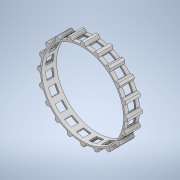
# Autodesk Inventor part: tracks_v1
Saved by Autodesk Inventor 2020 (Build 240168000, 168)
## iProperties
Created: 2020-04-20
Part Number: tracks_v1
Material: Ogólny
Document SubType Name: Modeling
Designer: blep
Density: 1 g/cm^3
Appearance: Domyślna
Author: blep
Autodesk Inventor part; units mm, degrees
ref_plane "XZ Plane" through (0, 0, 0) normal (0, 1, 0) x (-1, 0, 0)
ref_plane "XY Plane" through (0, 0, 0) normal (0, 0, 1) x (1, 0, 0)
sketch "Szkic1" plane through (0, 0, 0) normal (0, 0, 1) x (1, 0, 0)
  circle A0 centre (0, 0) radius 55.5545
  circle A1 centre (0, 0) radius 57.5545
  dimension "d0" = 111.109
  dimension "d1" = 2
  constraints: 2 centre point, 1 coincident
  measures "d0" diameter of A0
  measures "d1" radial gap between concentric circles of A0 A1
extrude "Wyciągnięcie proste1" add sketch "Szkic1" along normal blind 20
ref_plane "Płaszczyzna konstrukcyjna1" through (57.5545, 0, 0) normal (1, 0, 0) x (0, 1, 0)
sketch "Szkic2" plane through (57.5545, 0, 0) normal (1, 0, 0) x (0, 1, 0)
  line L0 (57.5545, 0) -> (-57.5545, 0)
  line L1 (57.5545, 20) -> (-57.5545, 20) projected
  line L2 (-3.764, 0) -> (3.764, 0)
  line L3 (3.764, 0) -> (3.764, 20)
  line L4 (3.764, 20) -> (-3.764, 20)
  line L5 (-3.764, 20) -> (-3.764, 0)
  line L6 (57.5545, 0) -> (-57.5545, 0) construction
  line L7 (-3.764, 20) -> (-57.5545, 0) construction
  line L8 (3.764, 20) -> (57.5545, 0) construction
  point P0 (-3.764, 20)
  point P1 (3.764, 0)
  dimension "d4" = 7.528
  constraints: 14 end point, 2 parallel, 1 equal length, 1 horizontal, 1 perpendicular, 1 point on line
  measures "d4" distance between parallel lines of L3 L5
extrude "Wyciągnięcie proste2" add sketch "Szkic2" along normal blind 4 and the other way blind 1
chamfer "Faza1" distance 2 distance2 4 1 edges at (61.5545, 3.764, 10) measured on face at (61.5545, 3.264, 10)
chamfer "Faza2" distance 2 distance2 4 1 edges at (61.5545, -3.764, 10) measured on face at (61.5545, -3.264, 10)
pattern_circular "Szyk kołowy1" count 20 over 360 about axis through (0, 0, 0) along (0, 0, 1) of "Wyciągnięcie proste2", "Faza1", "Faza2"
sketch "Szkic3" plane through (0, 0, 20) normal (0, 0, 1) x (1, 0, 0)
  line L0 (57.4313, -3.764) -> (55.4356, -3.6332)
  line L1 (55.7835, -14.1675) -> (53.8451, -13.6752)
  line L2 (0, 0) -> (57.4313, -3.764) construction
  line L3 (55.7835, -14.1675) -> (0, 0) construction
  arc A0 (53.8451, -13.6752) -> (55.4356, -3.6332) centre (0, 0) ccw
  arc A1 (55.7835, -14.1675) -> (57.4313, -3.764) centre (0, 0) ccw
  circle A2 centre (0, 0) radius 55.5545 construction
  line L4 (55.7835, 14.1675) -> (53.8451, 13.6752)
  line L5 (57.4313, 3.764) -> (55.4356, 3.6332)
  arc A3 (55.4356, 3.6332) -> (53.8451, 13.6752) centre (0, 0) ccw
  arc A4 (57.4313, 3.764) -> (55.7835, 14.1675) centre (0, 0) ccw
  line L6 (48.6753, 30.7121) -> (46.9839, 29.6449)
  line L7 (53.4573, 21.327) -> (51.5996, 20.5859)
  arc A5 (51.5996, 20.5859) -> (46.9839, 29.6449) centre (0, 0) ccw
  arc A6 (53.4573, 21.327) -> (48.6753, 30.7121) centre (0, 0) ccw
  line L8 (36.8024, 44.2505) -> (35.5235, 42.7128)
  line L9 (44.2505, 36.8024) -> (42.7128, 35.5235)
  arc A7 (42.7128, 35.5235) -> (35.5235, 42.7128) centre (0, 0) ccw
  arc A8 (44.2505, 36.8024) -> (36.8024, 44.2505) centre (0, 0) ccw
  line L10 (21.327, 53.4573) -> (20.5859, 51.5996)
  line L11 (30.7121, 48.6753) -> (29.6449, 46.9839)
  arc A9 (29.6449, 46.9839) -> (20.5859, 51.5996) centre (0, 0) ccw
  arc A10 (30.7121, 48.6753) -> (21.327, 53.4573) centre (0, 0) ccw
  line L12 (3.764, 57.4313) -> (3.6332, 55.4356)
  line L13 (14.1675, 55.7835) -> (13.6752, 53.8451)
  arc A11 (13.6752, 53.8451) -> (3.6332, 55.4356) centre (0, 0) ccw
  arc A12 (14.1675, 55.7835) -> (3.764, 57.4313) centre (0, 0) ccw
  line L14 (-14.1675, 55.7835) -> (-13.6752, 53.8451)
  line L15 (-3.764, 57.4313) -> (-3.6332, 55.4356)
  arc A13 (-3.6332, 55.4356) -> (-13.6752, 53.8451) centre (0, 0) ccw
  arc A14 (-3.764, 57.4313) -> (-14.1675, 55.7835) centre (0, 0) ccw
  line L16 (-30.7121, 48.6753) -> (-29.6449, 46.9839)
  line L17 (-21.327, 53.4573) -> (-20.5859, 51.5996)
  arc A15 (-20.5859, 51.5996) -> (-29.6449, 46.9839) centre (0, 0) ccw
  arc A16 (-21.327, 53.4573) -> (-30.7121, 48.6753) centre (0, 0) ccw
  line L18 (-44.2505, 36.8024) -> (-42.7128, 35.5235)
  line L19 (-36.8024, 44.2505) -> (-35.5235, 42.7128)
  arc A17 (-35.5235, 42.7128) -> (-42.7128, 35.5235) centre (0, 0) ccw
  arc A18 (-36.8024, 44.2505) -> (-44.2505, 36.8024) centre (0, 0) ccw
  line L20 (-53.4573, 21.327) -> (-51.5996, 20.5859)
  line L21 (-48.6753, 30.7121) -> (-46.9839, 29.6449)
  arc A19 (-46.9839, 29.6449) -> (-51.5996, 20.5859) centre (0, 0) ccw
  arc A20 (-48.6753, 30.7121) -> (-53.4573, 21.327) centre (0, 0) ccw
  line L22 (-57.4313, 3.764) -> (-55.4356, 3.6332)
  line L23 (-55.7835, 14.1675) -> (-53.8451, 13.6752)
  arc A21 (-53.8451, 13.6752) -> (-55.4356, 3.6332) centre (0, 0) ccw
  arc A22 (-55.7835, 14.1675) -> (-57.4313, 3.764) centre (0, 0) ccw
  line L24 (-55.7835, -14.1675) -> (-53.8451, -13.6752)
  line L25 (-57.4313, -3.764) -> (-55.4356, -3.6332)
  arc A23 (-55.4356, -3.6332) -> (-53.8451, -13.6752) centre (0, 0) ccw
  arc A24 (-57.4313, -3.764) -> (-55.7835, -14.1675) centre (0, 0) ccw
  line L26 (-48.6753, -30.7121) -> (-46.9839, -29.6449)
  line L27 (-53.4573, -21.327) -> (-51.5996, -20.5859)
  arc A25 (-51.5996, -20.5859) -> (-46.9839, -29.6449) centre (0, 0) ccw
  arc A26 (-53.4573, -21.327) -> (-48.6753, -30.7121) centre (0, 0) ccw
  line L28 (-36.8024, -44.2505) -> (-35.5235, -42.7128)
  line L29 (-44.2505, -36.8024) -> (-42.7128, -35.5235)
  arc A27 (-42.7128, -35.5235) -> (-35.5235, -42.7128) centre (0, 0) ccw
  arc A28 (-44.2505, -36.8024) -> (-36.8024, -44.2505) centre (0, 0) ccw
  line L30 (-21.327, -53.4573) -> (-20.5859, -51.5996)
  line L31 (-30.7121, -48.6753) -> (-29.6449, -46.9839)
  arc A29 (-29.6449, -46.9839) -> (-20.5859, -51.5996) centre (0, 0) ccw
  arc A30 (-30.7121, -48.6753) -> (-21.327, -53.4573) centre (0, 0) ccw
  line L32 (-3.764, -57.4313) -> (-3.6332, -55.4356)
  line L33 (-14.1675, -55.7835) -> (-13.6752, -53.8451)
  arc A31 (-13.6752, -53.8451) -> (-3.6332, -55.4356) centre (0, 0) ccw
  arc A32 (-14.1675, -55.7835) -> (-3.764, -57.4313) centre (0, 0) ccw
  line L34 (14.1675, -55.7835) -> (13.6752, -53.8451)
  line L35 (3.764, -57.4313) -> (3.6332, -55.4356)
  arc A33 (3.6332, -55.4356) -> (13.6752, -53.8451) centre (0, 0) ccw
  arc A34 (3.764, -57.4313) -> (14.1675, -55.7835) centre (0, 0) ccw
  line L36 (30.7121, -48.6753) -> (29.6449, -46.9839)
  line L37 (21.327, -53.4573) -> (20.5859, -51.5996)
  arc A35 (20.5859, -51.5996) -> (29.6449, -46.9839) centre (0, 0) ccw
  arc A36 (21.327, -53.4573) -> (30.7121, -48.6753) centre (0, 0) ccw
  line L38 (44.2505, -36.8024) -> (42.7128, -35.5235)
  line L39 (36.8024, -44.2505) -> (35.5235, -42.7128)
  arc A37 (35.5235, -42.7128) -> (42.7128, -35.5235) centre (0, 0) ccw
  arc A38 (36.8024, -44.2505) -> (44.2505, -36.8024) centre (0, 0) ccw
  line L40 (53.4573, -21.327) -> (51.5996, -20.5859)
  line L41 (48.6753, -30.7121) -> (46.9839, -29.6449)
  arc A39 (46.9839, -29.6449) -> (51.5996, -20.5859) centre (0, 0) ccw
  arc A40 (48.6753, -30.7121) -> (53.4573, -21.327) centre (0, 0) ccw
  point P0 (48.6753, 30.7121)
  point P1 (3.764, 57.4313)
  point P2 (-44.2505, 36.8024)
  point P3 (-53.4573, 21.327)
  point P4 (-55.7835, -14.1675)
  point P5 (-36.8024, -44.2505)
  point P6 (-21.327, -53.4573)
  point P7 (-3.764, -57.4313)
  point P8 (44.2505, -36.8024)
  point P9 (53.4573, -21.327)
  point P10 (57.4313, -3.764)
  dimension "d22" = 360
  constraints: 84 end point, 80 point on circle, 41 coincident, 40 centre point, 2 collinear, 2 point on line, 1 concentric, 221 other
extrude "Wyciągnięcie proste3" cut sketch "Szkic3" against normal blind 15
extrude "Wyciągnięcie proste4" add sketch "Szkic3" against normal blind 5
